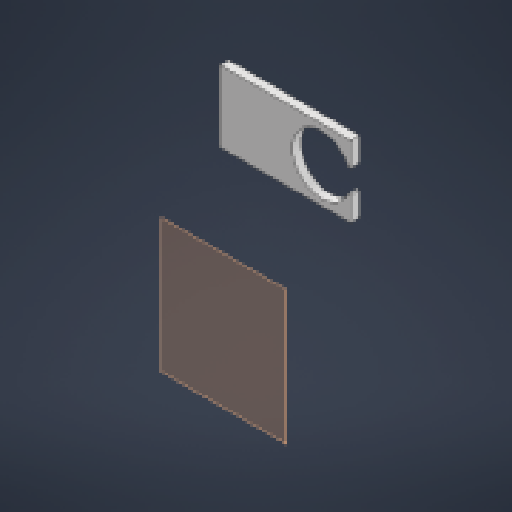
# Autodesk Inventor part: servo_holder
Saved by Autodesk Inventor 2024 (Build 280153000, 153)
## iProperties
Created: 2026-03-28
Part Number: servo_holder
Material: Generic
Document SubType Name: Modeling
Designer: schar
Density: 1 g/cm^3
Appearance: Default
Author: schar
Autodesk Inventor part; units mm, degrees
ref_plane "YZ Plane" through (0, 0, 0) normal (1, 0, 0) x (0, 1, 0)
ref_plane "XZ Plane" through (0, 0, 0) normal (0, 1, 0) x (-1, 0, 0)
ref_plane "XY Plane" through (0, 0, 0) normal (0, 0, 1) x (1, 0, 0)
ref_plane "Work Plane1" through (-30.9, -52.9315, 23.6) normal (0, 0, 1) x (0, -1, 0)
sketch "Sketch1" plane through (-30.9, -52.9315, 23.6) normal (0, 0, 1) x (0, -1, 0)
  circle A0 centre (-52.9315, 56.4) radius 1.3 projected
  circle A1 centre (-52.9315, 56.4) radius 9.6 projected
  line L0 (-65.1519, 50.7075) -> (-65.1519, 23.4294) projected
  line L1 (-65.2915, 23.2898) -> (-65.2915, 63.0172) projected
  arc A2 (-64.7058, 64.4313) -> (-65.2915, 63.0172) centre (-63.2917, 63.0172) ccw projected
  line L2 (-61.7987, 66.51) -> (-44.0643, 66.51) projected
  line L3 (-40.5715, 63.0172) -> (-40.5715, 23.2898) projected
  line L4 (-63.2933, 21.2883) -> (-42.5697, 21.2883) projected
  line L5 (-42.5697, 21.2883) -> (-37.8441, 21.2883)
  line L6 (-40.5715, 23.2898) -> (-40.5715, 18.074)
  line L7 (-63.2933, 21.2883) -> (-67.0577, 21.2883)
  line L8 (-65.2915, 23.2898) -> (-65.2915, 18.9646)
  line L9 (-65.2915, 63.0172) -> (-65.2915, 68.4057)
  line L10 (-61.7987, 66.51) -> (-67.4524, 66.51)
  line L11 (-40.5715, 63.0172) -> (-40.5715, 69.9342)
  line L12 (-44.0643, 66.51) -> (-38.7131, 66.51)
  circle A3 centre (-52.9315, 56.4) radius 10.1
  line L13 (-52.9315, 66.5) -> (-48.9315, 66.51)
  line L14 (-48.9315, 66.51) -> (-48.9294, 65.6733)
  line L15 (-52.9315, 66.5) -> (-56.9315, 66.51)
  line L16 (-56.9315, 66.51) -> (-56.9336, 65.6733)
  point P0 (-52.9315, 30.9)
  point P1 (-65.2915, 21.2883)
  point P2 (-40.5715, 21.2883)
  point P3 (-40.5715, 66.51)
  point P4 (-65.2915, 66.51)
  dimension "d0" = 20.2
  dimension "d1" = 4
  dimension "d2" = 4
  constraints: 24 end point, 3 horizontal, 3 perpendicular, 3 point on circle, 3 vertical, 2 point on line, 1 centre point, 1 coincident
  measures "d0" diameter of A3
  measures "d1" distance of L13.start L13.end
  measures "d2" distance of L13.start L15.end
extrude "Extrusion1" add sketch "Sketch1" along normal blind 3 contours L1 L9 L10 L2 L16 A3 L14 L12 L11 L3 L6 L5 L4 L7 L8
sketch "Sketch2" plane through (-30.9, -52.9315, 26.6) normal (0, 0, 1) x (1, 0, 0)
  circle A0 centre (81.5325, 36.2648) radius 2.15 projected
  circle A1 centre (91.5325, 18.9443) radius 2.15 projected
  line L0 (80.8626, 47.4251) -> (72.2024, 42.4251) projected
  line L1 (80.8626, 47.4251) -> (100.8626, 12.7841) projected
  line L2 (92.2024, 7.7841) -> (100.8626, 12.7841) projected
  line L3 (72.2024, 42.4251) -> (92.2024, 7.7841) projected
  circle A2 centre (58.2675, 83.0302) radius 2.15 projected
  circle A3 centre (68.2675, 100.3507) radius 2.15 projected
  line L4 (48.9374, 76.87) -> (57.5976, 71.87) projected
  line L5 (48.9374, 76.87) -> (68.9374, 111.511) projected
  line L6 (77.5976, 106.511) -> (68.9374, 111.511) projected
  line L7 (57.5976, 71.87) -> (77.5976, 106.511) projected
  circle A4 centre (29.4, 39.6495) radius 2.15 projected
  circle A5 centre (9.4, 39.6495) radius 2.15 projected
  line L8 (39.4, 34.6495) -> (39.4, 44.6495) projected
  line L9 (39.4, 34.6495) -> (-0.6, 34.6495) projected
  line L10 (-0.6, 44.6495) -> (-0.6, 34.6495) projected
  line L11 (39.4, 44.6495) -> (-0.6, 44.6495) projected
  line L12 (48.9374, 76.87) -> (42.2526, 65.2915)
  line L13 (66.51, 65.2915) -> (21.2883, 65.2915) projected
  line L14 (57.5976, 71.87) -> (53.7996, 65.2915)
  line L15 (72.2024, 42.4251) -> (66.51, 42.4251)
  line L16 (66.51, 40.5715) -> (66.51, 48.9315) projected
  line L17 (80.8626, 47.4251) -> (76.0949, 48.9315)
  line L18 (76.0949, 48.9315) -> (66.51, 48.9315)
  line L19 (19.4, 44.6495) -> (19.4, 34.6495)
  line L20 (-0.6, 44.6495) -> (21.2883, 65.2915)
  line L21 (19.4, 44.6495) -> (21.2883, 46.4303)
  line L22 (21.2883, 65.2915) -> (21.2883, 40.5715) projected
  point P0 (30.9, 52.9315)
  dimension "d5" = 5
  constraints: 16 end point, 4 point on line, 2 collinear, 2 horizontal, 2 midpoint, 1 parallel
  measures "d5" distance of L0.start L17.end
ref_plane "Work Plane2" through (8.0374, 16.4384, 38.8317) normal (0, 0, -1) x (0.5, 0.8660254, 0)
extrude "Extrusion2" add sketch "Sketch2" along normal up to surface (12.2317 mm away) contours L1 L2 L3 L0 | L0 L15 L16 L18 L17 | L5 L6 L7 L4 | L4 L14 L13 L12 | L9 L10 L11 L19 | L11 L20 L22 L21
sketch "Sketch3" plane through (-31.5, -18.282, 38.8317) normal (0, 0, 1) x (1, 0, 0)
  circle A0 centre (30, 5) radius 2.15 projected
  circle A1 centre (10, 5) radius 2.15 projected
  line L0 (40, 0) -> (40, 10) projected
  line L1 (40, 0) -> (0, 0) projected
  line L2 (0, 10) -> (0, 0) projected
  line L3 (40, 10) -> (0, 10) projected
  line L4 (20, 0) -> (20, 10) projected
  line L5 (20, 0) -> (20, 10)
  point P0 (31.5, 18.282)
  constraints: 2 end point, 1 midpoint, 1 vertical
extrude "Extrusion3" add sketch "Sketch3" against normal blind 4 contours L1 L4 L3 L0
sketch "Sketch4" plane through (35.61, 4, 23.6) normal (1, 0, 0) x (0, 0, -1)
  line L0 (-3, 8.36) -> (0, 8.36)
  line L1 (0, 8.36) -> (0, -16.36)
  line L2 (0, -16.36) -> (-3, -16.36)
  line L3 (-3, -16.36) -> (-3, 8.36)
  point P0 (23.6, -4)
  constraints: 8 end point, 2 parallel, 1 horizontal, 1 perpendicular
extrude "Extrusion4" add sketch "Sketch4" along normal blind 10
sketch "Sketch5" plane through (45.61, 4, 23.6) normal (1, 0, 0) x (0, 0, -1)
  line L0 (-3, -8) -> (-15.2317, -8) projected
  line L1 (-3, 8.36) -> (-3, -8.1311) projected
  line L2 (-15.2317, -8) -> (-3, 8.36)
  point P0 (23.6, -4)
  constraints: 2 end point
extrude "Extrusion5" add sketch "Sketch5" against normal up to surface (10 mm away)
sketch "Sketch6" plane through (38.0374, 58.5795, 26.6) normal (-0.8660254, 0.5, 0) x (0, 0, 1)
  line L0 (0, -53.3696) -> (0, -63.8518) projected
  line L1 (0, -53.3696) -> (0, -65.3696)
  line L2 (12.2317, 0) -> (12.2317, -53.3696) projected
  line L3 (0, -65.3696) -> (12.2317, -53.3696)
  line L4 (0, -53.3696) -> (12.2317, -53.3696) projected
  line L5 (0, -47.5961) -> (12.2317, -47.5961) projected
  line L6 (0, 0) -> (0, -53.3696) projected
  point P0 (-26.6, -69.75)
  point P1 (49.125, -56.6968)
  point P2 (0, -63.8518)
  dimension "d14" = 12
  constraints: 4 end point, 1 collinear, 1 other
  measures "d14" distance of L0.start L1.end
extrude "Extrusion6" add sketch "Sketch6" against normal blind 10
sketch "Sketch7" plane through (-9.6117, 12.36, 26.6) normal (0, 1, 0) x (1, 0, 0)
  line L0 (0, 0) -> (0, -12.2317) projected
  line L1 (0, -12.2317) -> (11.8061, 0)
  line L2 (0, 0) -> (51.9842, 0) projected
  line L3 (0, 3) -> (0, 0) projected
  line L4 (11.8061, 0) -> (0, 0)
  point P0 (9.6117, 26.6)
  dimension "d17" = 17
  constraints: 4 end point, 1 perpendicular, 1 point on line
  measures "d17" distance of L0.end L1.end
extrude "Extrusion7" add sketch "Sketch7" against normal up to surface surface through (-11.5, -8.282, 26.6) normal (0.686092, -0.7275148, 0)
sketch "Sketch8" plane through (-30.9, -52.9315, 23.6) normal (0, 0, -1) x (-1, 0, 0)
  circle A0 centre (-23.65, 63.1815) radius 1
  circle A1 centre (-23.65, 42.6815) radius 0.8
  circle A2 centre (-23.65, 63.1815) radius 0.8
  circle A3 centre (-48.1, 42.6815) radius 0.8
  circle A4 centre (-27.4, 42.6815) radius 0.8
  circle A5 centre (-27.4, 63.1815) radius 0.8
  circle A6 centre (-48.1, 63.1815) radius 0.8
  point P0 (-30.9, 52.9315)
extrude "Extrusion8" cut sketch "Sketch8" against normal through all contours A1 | A2 | A3 | A4 | A5 | A6
sketch "Sketch9" plane through (-30.9, -52.9315, 23.6) normal (0, 0, -1) x (-1, 0, 0)
  point P0 (-30.9, 52.9315)
sketch "Sketch10" plane through (-9.6117, -12.36, 23.6) normal (-1, 0, 0) x (0, 0, 1)
  line L0 (-1.1, 2.36) -> (-1.1, 0.9818) projected
  line L1 (-1.1, 5.36) -> (-0.2134, 5.4376) projected
  line L2 (-0.2134, 19.2824) -> (-1.1, 19.36) projected
  line L3 (-1.1, 20.21) -> (-1.1, 22.36) projected
  line L4 (-1.1, 23.7382) -> (-1.1, 22.36) projected
  line L5 (-1.1, 2.36) -> (-1.1, 4.51) projected
  line L6 (-1.1, 5.3728) -> (-1.1, 4.51) projected
  line L7 (-1.1, 20.21) -> (-1.1, 19.3472) projected
  line L8 (0, 22.46) -> (0, 2.26) projected
  line L9 (-1.1, 5.3728) -> (-1.1, 0.9818)
  line L10 (0, 0) -> (-1.1, 0)
  line L11 (-1.1, 0) -> (-1.1, 0.9818)
  line L12 (-1.1, 5.36) -> (0, 5.4562)
  line L13 (0, 0) -> (0, 5.4562)
  line L14 (-1.1, 19.36) -> (0, 19.2638)
  line L15 (0, 0) -> (0, 24.72) projected
  line L16 (0, 19.2638) -> (0, 24.72)
  line L17 (0, 24.72) -> (-1.1, 24.72)
  line L18 (-1.1, 24.72) -> (-1.1, 19.36)
  line L19 (-0.9176, 19.344) -> (-0.9089, 19.444)
  line L20 (-1.3675, 19.4842) -> (0.1907, 19.3478)
  line L21 (-0.6159, 5.4023) -> (-0.6072, 5.3023)
  line L22 (-1.5011, 5.2241) -> (0.1823, 5.3714)
  point P0 (-23.6, 12.36)
  point P1 (0, 8.3579)
  point P2 (0, 16.3621)
  point P3 (0, 2.26)
  point P4 (0, 5.3555)
  point P5 (-1.1, 5.2592)
  point P6 (-1.1, 19.4608)
  point P7 (0, 19.3645)
  dimension "d22" = 0.1
  dimension "d23" = 0.1
  constraints: 26 end point, 8 point on line, 6 perpendicular, 3 collinear, 2 vertical, 1 parallel
  measures "d22" vertical distance of L19.end L19.start
  measures "d23" vertical distance of L21.start L21.end
extrude "Extrusion9" add sketch "Sketch10" against normal up to surface (45.2217 mm away) contours L5 L6 L22 L8 L13 L10 L11 L0 | L20 L7 L3 L4 L18 L17 L15 L8
sketch "Sketch11" plane through (-30.9, -52.9315, 26.6) normal (0, 0, 1) x (1, 0, 0)
  circle A0 centre (48.1, 42.6815) radius 0.8 projected
  circle A1 centre (27.4, 42.6815) radius 0.8 projected
  circle A2 centre (23.65, 42.6815) radius 0.8 projected
  circle A3 centre (23.65, 63.1815) radius 0.8 projected
  circle A4 centre (27.4, 63.1815) radius 0.8 projected
  circle A5 centre (48.1, 63.1815) radius 0.8 projected
  point P0 (30.9, 52.9315)
extrude "Extrusion10" cut sketch "Sketch11" against normal through all
sketch "Sketch12" plane through (-31.5, -18.282, 34.8317) normal (0, 0, -1) x (-1, 0, 0)
  circle A0 centre (-28, 8.032) radius 0.8 projected
  circle A1 centre (-24.25, 8.032) radius 0.8 projected
  line L0 (-20, 10) -> (-40, 10) projected
  line L1 (-40, 10) -> (-40, 0) projected
  line L2 (-40, 0) -> (-20, 0) projected
  line L3 (-20, 10) -> (-20, 0) projected
  circle A2 centre (-30, 5) radius 2.15 projected
  point P0 (-31.5, 18.282)
ref_plane "Work Plane3" through (-35.8301, -35.6025, 38.9818) normal (0, 0, -1) x (0, 1, 0)
extrude "Extrusion11" add sketch "Sketch12" against normal up to surface (4.15 mm away) contours A0 | A1
sketch "Sketch13" plane through (-9.6117, -12.36, 22.5) normal (0, 0, -1) x (-1, 0, 0)
  circle A0 centre (-35.1117, 12.36) radius 1.3 projected
  circle A1 centre (-35.1117, 12.36) radius 10.1
  point P0 (-9.6117, 12.36)
  constraints: 1 centre point, 1 coincident
extrude "Extrusion12" cut sketch "Sketch13" against normal through all
body "Solid1"
